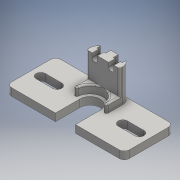
# Autodesk Inventor part: plate
Saved by Autodesk Inventor 2016 (Build 200138000, 138)
## iProperties
Created: 2016-02-21
Part Number: plate
Material: Generic
Document SubType Name: Modeling
Designer: Mikkel
Density: 1 g/cm^3
Appearance: Default
Author: Mikkel
Autodesk Inventor part; units mm, degrees
ref_plane "YZ Plane" through (0, 0, 0) normal (1, 0, 0) x (0, 1, 0)
ref_plane "XZ Plane" through (0, 0, 0) normal (0, 1, 0) x (-1, 0, 0)
ref_plane "XY Plane" through (0, 0, 0) normal (0, 0, 1) x (1, 0, 0)
sketch "Sketch1" plane through (0, 0, 0) normal (0, 0, 1) x (1, 0, 0)
  line L0 (0, 0) -> (71.6, 0)
  line L1 (71.6, 0) -> (71.6, 29.85)
  line L2 (71.6, 29.85) -> (0, 29.85)
  line L3 (0, 29.85) -> (0, 0)
  circle A0 centre (35.8, 14.925) radius 6.1
  line L4 (29.7, 0) -> (29.7, 14.925)
  line L5 (41.9, 0) -> (41.9, 14.925)
  circle A1 centre (15.8, 14.925) radius 2.8
  circle A2 centre (5.8, 14.925) radius 2.8
  circle A3 centre (55.8, 14.925) radius 2.8
  circle A4 centre (65.8, 14.925) radius 2.8
  line L6 (5.8, 17.725) -> (15.8, 17.725)
  line L7 (5.8, 12.125) -> (15.8, 12.125)
  line L8 (55.8, 17.725) -> (65.8, 17.725)
  line L9 (55.8, 12.125) -> (65.8, 12.125)
  dimension "d0" = 71.6
  dimension "d1" = 29.85
  dimension "d2" = 12.2
  dimension "d3" = 5.8
  dimension "d4" = 15.8
  dimension "d5" = 55.8
  dimension "d6" = 65.8
  dimension "d7" = 5.6
  dimension "d8" = 5.6
  dimension "d9" = 5.6
  dimension "d10" = 5.6
  dimension "d11" = 14.925
  dimension "d12" = 14.925
  dimension "d13" = 14.925
  dimension "d14" = 14.925
  constraints: 20 end point, 10 point on circle, 10 tangent, 5 centre point, 3 perpendicular, 2 parallel, 2 point on line, 1 horizontal, 1 other
  measures "d0" distance of L2.end L1.end
  measures "d1" distance of L1.end L0.end
  measures "d2" diameter of A0
  measures "d3" distance from line of L3 A2.centre
  measures "d4" distance from line of L3 A1.centre
  measures "d5" distance from line of L3 A3.centre
  measures "d6" distance from line of A4.centre L3
  measures "d7" diameter of A2
  measures "d8" diameter of A1
  measures "d9" diameter of A3
  measures "d10" diameter of A4
  measures "d11" distance from line of L0 A3.centre
  measures "d12" distance from line of L0 A4.centre
  measures "d13" distance from line of L0 A2.centre
  measures "d14" distance from line of L0 A1.centre
extrude "Extrusion1" add sketch "Sketch1" along normal blind 4.6 contours L3 L2 L1 L0 L5 A0 L4
fillet "Fillet1" radius 3 4 edges at (71.6, 29.85, 2.3) (0, 29.85, 2.3) (0, 0, 2.3) (71.6, 0, 2.3)
sketch "Sketch2" plane through (0, 0, 4.6) normal (0, 0, 1) x (1, 0, 0)
  line L0 (25.8, 29.85) -> (45.8, 29.85)
  line L1 (45.8, 29.85) -> (45.8, 22.925)
  line L2 (45.8, 22.925) -> (25.8, 22.925)
  line L3 (25.8, 22.925) -> (25.8, 29.85)
  arc A0 (41.9, 14.925) -> (29.7, 14.925) centre (35.8, 14.925) ccw projected
  line L4 (68.6, 29.85) -> (3, 29.85) projected
  circle A1 centre (35.8, 14.925) radius 8
  line L5 (25.8, 22.925) -> (25.8, 14.925)
  line L6 (25.8, 14.925) -> (27.8, 14.925)
  line L7 (45.8, 22.925) -> (45.8, 14.925)
  line L8 (45.8, 14.925) -> (43.8, 14.925)
  point P0 (0, 0)
  point P1 (35.8, 22.925)
  dimension "d18" = 20
  dimension "d19" = 10
  dimension "d23" = 16
  constraints: 16 end point, 3 point on circle, 2 coincident, 2 parallel, 2 perpendicular, 2 point on line, 1 centre point, 1 collinear, 1 horizontal, 1 midpoint, 1 vertical
  measures "d18" distance of L0.start L0.end
  measures "d19" distance from line of L3 point (35.8, 14.925)
  measures "d23" diameter of A1
extrude "Extrusion2" add sketch "Sketch2" along normal blind 20 contours L0 L1 L2 L3
extrude "Extrusion3" add sketch "Sketch2" along normal blind 5 contours L2 A1 L6 L5 | L7 L8 A1 L2
fillet "Fillet2" radius 1 12 edges at (25.8, 14.925, 7.1) (27.8, 14.925, 7.1) (43.8, 14.925, 7.1) (45.8, 14.925, 7.1) (25.8, 18.925, 9.6) (26.8, 14.925, 9.6) (30.1431, 20.5819, 9.6) (41.4569, 20.5819, 9.6) (44.8, 14.925, 9.6) (45.8, 18.925, 9.6) (25.8, 22.925, 17.1) (45.8, 22.925, 17.1)
fillet "Fillet3" radius 5 2 edges at (25.8, 29.85, 14.6) (45.8, 29.85, 14.6)
sketch "Sketch3" plane through (26.8, 22.925, 24.6) normal (0, -1, 0) x (1, 0, 0)
  circle A0 centre (4, -2.4) radius 1.6
  circle A1 centre (14, -2.4) radius 1.6
  line L0 (0, 0) -> (18, 0) projected
  line L1 (-1, 0) -> (-1, -16) projected
  line L2 (19, -16) -> (19, 0) projected
  line L3 (2.4, -2.4) -> (2.4, 0)
  line L4 (5.6, -2.4) -> (5.6, 0)
  line L5 (12.4, -2.4) -> (12.4, 0)
  line L6 (15.6, -2.4) -> (15.6, 0)
  point P0 (-26.8, -24.6)
  dimension "d30" = 5
  dimension "d31" = 5
  dimension "d38" = 4
  dimension "d39" = 3.2
  dimension "d40" = 3.2
  dimension "d41" = 4
  constraints: 8 end point, 4 point on circle, 4 point on line, 4 tangent, 3 perpendicular, 2 centre point, 1 parallel
  measures "d30" distance from line of L1 A0.centre
  measures "d31" distance from line of L2 A1.centre
  measures "d39" diameter of A0
  measures "d40" diameter of A1
extrude "Extrusion4" cut sketch "Sketch3" against normal through all
sketch "Sketch4" plane through (3, 29.85, 0) normal (0, 1, 0) x (1, 0, 0)
  circle A0 centre (37.8, -22.2) radius 1.6 projected
  line L0 (35.0718, -20.5751) -> (37.8431, -19.0249)
  line L1 (37.8431, -19.0249) -> (40.5713, -20.6497)
  line L2 (40.5713, -20.6497) -> (40.5282, -23.8249)
  line L3 (40.5282, -23.8249) -> (37.7569, -25.3751)
  line L4 (37.7569, -25.3751) -> (35.0287, -23.7503)
  line L5 (35.0287, -23.7503) -> (35.0718, -20.5751)
  circle A1 centre (27.8, -22.2) radius 1.6 projected
  line L6 (30.55, -23.7877) -> (27.8, -25.3754)
  line L7 (27.8, -25.3754) -> (25.05, -23.7877)
  line L8 (25.05, -23.7877) -> (25.05, -20.6123)
  line L9 (25.05, -20.6123) -> (27.8, -19.0246)
  line L10 (27.8, -19.0246) -> (30.55, -20.6123)
  line L11 (30.55, -20.6123) -> (30.55, -23.7877)
  line L12 (40.5282, -23.8249) -> (40.5282, -24.6)
  line L13 (40.5282, -24.6) -> (39.1426, -24.6)
  line L14 (35.0287, -23.7503) -> (35.0287, -24.6)
  line L15 (29.4, -24.6) -> (36.2, -24.6) projected
  line L16 (35.0287, -24.6) -> (36.4555, -24.6)
  line L17 (30.55, -23.7877) -> (30.55, -24.6)
  line L18 (30.55, -24.6) -> (29.1431, -24.6)
  line L19 (39.4, -24.6) -> (41.8, -24.6) projected
  line L20 (25.05, -23.7877) -> (25.05, -24.6)
  line L21 (23.8, -24.6) -> (26.2, -24.6) projected
  line L22 (25.05, -24.6) -> (26.4569, -24.6)
  point P0 (-3, 0)
  dimension "d34" = 5.5
  dimension "d35" = 5.5
  constraints: 40 end point, 7 point on line, 3 collinear, 2 coincident, 2 perpendicular, 2 vertical, 1 midpoint, 26 other
  measures "d34" distance between parallel lines of L2 L5
  measures "d35" distance between parallel lines of L8 L11
extrude "Extrusion5" cut sketch "Sketch4" against normal blind 3
body "Solid1"
